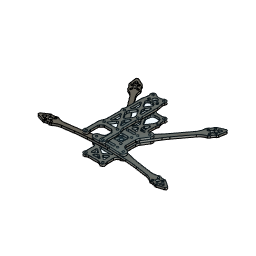
3inch Frame M3 v4 (Autodesk Fusion 360 design; units mm, degrees)
Autodesk Fusion 360 part; units mm, degrees
(part 1 of 3)
sketch "Skizze1" plane through (0, 0, 0) normal (0, 0, 1) x (1, 0, 0)
  line L0 (-8.4986, -15.4937) -> (8.4986, -15.4937)
  arc A0 (-5, -8.5) -> (-5, -11.5) centre (-5, -10) ccw
  line L1 (5.5, 1.5) -> (5.5, 8.5)
  arc A1 (-2.5, 11.5) -> (-5.5, 8.5) centre (-2.5, 8.5) ccw
  line L2 (9.0781, -17.3087) -> (1.159, -22.94)
  line L3 (-5, 18.5) -> (5, 18.5)
  arc A2 (5.5, 8.5) -> (2.5, 11.5) centre (2.5, 8.5) ccw
  line L4 (4.5469, -30.6788) -> (1.159, -28.2697)
  arc A3 (-16.0602, -5.4602) -> (-15.2136, -4.7566) centre (-25.2187, 6.4193) ccw
  line L5 (8.4205, -21.4575) -> (3.7344, -24.7899)
  line L6 (3.7344, -26.4198) -> (8.4205, -29.7522)
  circle A4 centre (12.5, -34.4937) radius 1
  arc A5 (-15.2136, -4.7566) -> (-13.8136, -1.2866) centre (-18.8136, -1.2866) ccw
  line L7 (5, 21.5) -> (-5, 21.5)
  arc A6 (1.159, -22.94) -> (-1.159, -22.94) centre (0, -21.3101) cw
  arc A7 (-9.6254, 27.8499) -> (-2.1571, 24.5) centre (-2.1571, 34.5) ccw
  line L8 (-5.5, 8.5) -> (-5.5, 1.5)
  circle A8 centre (-17.7913, 30.4065) radius 1
  arc A9 (11.2528, -36.6604) -> (8.7583, -35.9937) centre (8.7583, -40.9937) ccw
  line L9 (-5, -11.5) -> (5, -11.5)
  line L10 (-1.159, -28.2697) -> (-4.5469, -30.6788)
  arc A10 (2.5, -1.5) -> (5.5, 1.5) centre (2.5, 1.5) ccw
  line L11 (-1.159, -22.94) -> (-9.0781, -17.3087)
  arc A11 (1.159, -28.2697) -> (-1.159, -28.2697) centre (0, -29.8996) ccw
  arc A12 (-21.5229, 28.0783) -> (-14.5065, 33.3315) centre (-17.7913, 30.4065) cw
  arc A13 (-5.5, 1.5) -> (-2.5, -1.5) centre (-2.5, 1.5) ccw
  line L12 (-8.4205, -29.7522) -> (-3.7344, -26.4198)
  arc A14 (-10, -28.9372) -> (-8.4205, -29.7522) centre (-9, -28.9372) ccw
  line L13 (-15, -34.4937) -> (-15, -21.0235)
  line L14 (-13.8136, -1.2866) -> (-13.8136, 12.8582)
  arc A15 (5, -11.5) -> (5, -8.5) centre (5, -10) ccw
  line L15 (-14.5065, 33.3315) -> (-9.6254, 27.8499)
  line L16 (-2.5, -1.5) -> (2.5, -1.5)
  line L17 (5, -8.5) -> (-5, -8.5)
  arc A16 (3.9674, -32.4937) -> (4.5469, -30.6788) centre (3.9674, -31.4937) ccw
  line L18 (-3.9674, -32.4937) -> (3.9674, -32.4937)
  arc A17 (8.4986, -15.4937) -> (9.0781, -17.3087) centre (8.4986, -16.4937) cw
  line L19 (-3.7344, -24.7899) -> (-8.4205, -21.4575)
  arc A18 (-9.0781, -17.3087) -> (-8.4986, -15.4937) centre (-8.4986, -16.4937) cw
  line L20 (15, -21.0235) -> (15, -34.4937)
  arc A19 (19.9477, -16.0238) -> (15, -21.0235) centre (20, -21.0235) ccw
  arc A20 (8.4205, -29.7522) -> (10, -28.9372) centre (9, -28.9372) ccw
  line L21 (2.5, 11.5) -> (-2.5, 11.5)
  arc A21 (-4.5469, -30.6788) -> (-3.9674, -32.4937) centre (-3.9674, -31.4937) ccw
  arc A22 (15, -34.4937) -> (11.2528, -36.6604) centre (12.5, -34.4937) cw
  line L22 (13.8136, 12.8582) -> (13.8136, -1.2866)
  arc A23 (5, 18.5) -> (5, 21.5) centre (5, 20) ccw
  line L23 (-2.1571, 24.5) -> (2.1571, 24.5)
  circle A24 centre (-8, 13) radius 2
  arc A25 (15.3294, 18.1516) -> (13.8136, 12.8582) centre (23.8136, 12.8582) ccw
  circle A26 centre (-10, -10) radius 1
  arc A27 (10, -22.2725) -> (8.4205, -21.4575) centre (9, -22.2725) ccw
  circle A28 centre (19.8995, -11.4142) radius 1
  line L24 (8.7583, -35.9937) -> (-8.7583, -35.9937)
  line L25 (21.5229, 28.0783) -> (15.3294, 18.1516)
  arc A29 (-8.4205, -21.4575) -> (-10, -22.2725) centre (-9, -22.2725) ccw
  circle A30 centre (10, 20) radius 1
  arc A31 (-11.2528, -36.6604) -> (-15, -34.4937) centre (-12.5, -34.4937) cw
  arc A32 (-5, 21.5) -> (-5, 18.5) centre (-5, 20) ccw
  arc A33 (-3.7344, -26.4198) -> (-3.7344, -24.7899) centre (-4.3139, -25.6048) ccw
  arc A34 (-13.8136, 12.8582) -> (-15.3294, 18.1516) centre (-23.8136, 12.8582) ccw
  arc A35 (-17.6687, -6.1538) -> (-16.0602, -5.4602) centre (-18.8136, -1.2866) ccw
  line L26 (10, -28.9372) -> (10, -22.2725)
  arc A36 (20.9551, -6.9268) -> (19.9477, -16.0238) centre (19.8995, -11.4142) cw
  arc A37 (-8.7583, -35.9937) -> (-11.2528, -36.6604) centre (-8.7583, -40.9937) ccw
  circle A38 centre (8, 13) radius 2
  arc A39 (3.7344, -24.7899) -> (3.7344, -26.4198) centre (4.3139, -25.6048) ccw
  arc A40 (-15, -21.0235) -> (-19.9477, -16.0238) centre (-20, -21.0235) ccw
  arc A41 (-19.9477, -16.0238) -> (-20.9551, -6.9268) centre (-19.8995, -11.4142) cw
  arc A42 (15.2136, -4.7566) -> (16.0602, -5.4602) centre (25.2187, 6.4193) ccw
  circle A43 centre (10, -10) radius 1
  line L27 (9.6254, 27.8499) -> (14.5065, 33.3315)
  arc A44 (14.5065, 33.3315) -> (21.5229, 28.0783) centre (17.7913, 30.4065) cw
  line L28 (-15.3294, 18.1516) -> (-21.5229, 28.0783)
  circle A45 centre (-10, 20) radius 1
  circle A46 centre (8, -3) radius 2
  line L29 (17.6687, -6.1538) -> (20.9551, -6.9268)
  circle A47 centre (-19.8995, -11.4142) radius 1
  line L30 (-10, -22.2725) -> (-10, -28.9372)
  arc A48 (16.0602, -5.4602) -> (17.6687, -6.1538) centre (18.8136, -1.2866) ccw
  arc A49 (2.1571, 24.5) -> (9.6254, 27.8499) centre (2.1571, 34.5) ccw
  circle A50 centre (17.7913, 30.4065) radius 1
  circle A51 centre (-8, -3) radius 2
  arc A52 (13.8136, -1.2866) -> (15.2136, -4.7566) centre (18.8136, -1.2866) ccw
  circle A53 centre (-12.5, -34.4937) radius 1
  line L31 (-20.9551, -6.9268) -> (-17.6687, -6.1538)
extrude "Extrusion1" add sketch "Skizze1" along normal blind 3 makes body 1
sketch "Skizze2" plane through (0, 0, 0) normal (0, 0, 1) x (1, 0, 0)
  line L0 (50, -34.4937) -> (50, -19.2343)
  line L1 (25, -34.4937) -> (25, -14.0047)
  line L2 (28, 23.7417) -> (28, 48.0166)
  line L3 (28, 48.0166) -> (29.8264, 57.6051)
  arc A0 (30.5876, -17.771) -> (30, -19.187) centre (32, -19.187) ccw
  arc A1 (28, 16.2583) -> (27.3032, 18.6637) centre (23.5, 16.2583) ccw
  arc A2 (29.6382, 60.1802) -> (32.8799, 63.34) centre (32, 61) cw
  arc A3 (32.8799, 63.34) -> (33.9859, 62.9958) centre (36.3995, 72.7002) ccw
  arc A4 (46.584, -14.9827) -> (45.1731, -14.3952) centre (45.168, -16.3952) ccw
  arc A5 (34.8299, -14.3692) -> (33.4124, -14.9532) centre (34.8249, -16.3692) ccw
  line L4 (28, -3.4691) -> (28, 16.2583)
  arc A6 (37.582, 62.1014) -> (42.4175, 62.1034) centre (39.9957, 71.8057) ccw
  line L5 (42.4175, 62.1034) -> (46.0651, 63.0139)
  arc A7 (25, -14.0047) -> (26.5, -8.7369) centre (35, -14.0047) cw
  line L6 (45.1731, -14.3952) -> (34.8299, -14.3692)
  arc A8 (27.3032, 21.3363) -> (28, 23.7417) centre (23.5, 23.7417) ccw
  arc A9 (30, -34.4937) -> (25, -34.4937) centre (27.5, -34.4937) cw
  line L7 (33.9859, 62.9958) -> (37.582, 62.1014)
  arc A10 (27.3032, 18.6637) -> (27.3032, 21.3363) centre (29.4161, 20) cw
  line L8 (49.416, -17.8218) -> (46.584, -14.9827)
  arc A11 (52, -3.4691) -> (53.5, -8.7369) centre (62, -3.4691) ccw
  line L9 (37.0465, 33.3303) -> (37.0465, 35.9896)
  arc A12 (50, -19.2343) -> (49.416, -17.8218) centre (48, -19.2343) ccw
  line L10 (33.4124, -14.9532) -> (30.5876, -17.771)
  arc A13 (29.8264, 57.6051) -> (29.6382, 60.1802) centre (24.9147, 58.5407) ccw
  arc A14 (26.5, -8.7369) -> (28, -3.4691) centre (18, -3.4691) ccw
  line L11 (30, -19.187) -> (30, -34.4937)
  arc A15 (41.1255, 30.2175) -> (40.2838, 30.6775) centre (40.2838, 29.6775) ccw
  line L12 (34.1057, -9.3447) -> (45.9091, -9.3743)
  arc A16 (50.3618, 60.1802) -> (50.1736, 57.6051) centre (55.0853, 58.5407) ccw
  arc A17 (37.0465, 35.9896) -> (36.7299, 37.0695) centre (35.0465, 35.9896) ccw
  arc A18 (45.9091, -9.3743) -> (46.7436, -7.8196) centre (45.9116, -8.3743) ccw
  circle A19 centre (40, 56) radius 3.5
  arc A20 (33.3417, 42.3511) -> (31.5, 41.8112) centre (32.5, 41.8112) ccw
  arc A21 (36.3941, 50.4723) -> (38.2518, 50.7852) centre (37.6161, 48.889) cw
  arc A22 (52.6968, 18.6637) -> (52, 16.2583) centre (56.5, 16.2583) ccw
  line L13 (31.5, 38.4821) -> (31.6182, 27.626)
  arc A23 (38.2518, 50.7852) -> (41.7506, 50.7861) centre (40, 56) ccw
  arc A24 (45.3088, 49.1634) -> (45.7766, 46.5077) centre (44.0879, 47.5793) cw
  arc A25 (32.8235, 54.192) -> (34.7612, 54.3251) centre (33.8087, 54.0206) cw
  arc A26 (38.3359, 10.2003) -> (41.6641, 10.2003) centre (40, 11.3097) ccw
  arc A27 (39.8091, 38.6775) -> (38.9674, 39.1376) centre (39.8091, 39.6775) cw
  arc A28 (39.8347, 30.6775) -> (38.9903, 30.2133) centre (39.8347, 29.6775) ccw
  line L14 (45.7766, 46.5077) -> (41.1027, 39.1418)
  arc A29 (45.8881, 51.4617) -> (47.4838, 52.4251) centre (46.4986, 52.2538) ccw
  arc A30 (41.7506, 50.7861) -> (43.6082, 50.4741) centre (42.3872, 48.8901) cw
  circle A31 centre (50, -10) radius 1
  arc A32 (41.6641, -0.2003) -> (38.3359, -0.2003) centre (40, -1.3097) ccw
  arc A33 (33.2761, -7.79) -> (34.1057, -9.3447) centre (34.1082, -8.3447) ccw
  line L15 (46.168, 22.3571) -> (41.1255, 30.2175)
  arc A34 (46.0651, 63.0139) -> (47.1287, 63.3432) centre (43.6434, 72.7162) ccw
  arc A35 (36.7352, 32.2588) -> (37.0465, 33.3303) centre (35.0465, 33.3303) ccw
  line L16 (46.7436, -7.8196) -> (41.6641, -0.2003)
  line L17 (38.9903, 30.2133) -> (33.9075, 22.203)
  line L18 (34.7032, 49.1673) -> (36.3941, 50.4723)
  arc A36 (34.7612, 54.3251) -> (35.1808, 53.3495) centre (40, 56) ccw
  line L19 (52, 16.2583) -> (52, -3.4691)
  line L20 (38.3359, -0.2003) -> (33.2761, -7.79)
  arc A37 (33.9075, 22.203) -> (33.969, 16.7506) centre (38.1293, 19.5241) ccw
  line L21 (47.4838, 52.4251) -> (47.1765, 54.192)
  line L22 (52, 48.0166) -> (52, 23.7417)
  line L23 (33.969, 16.7506) -> (38.3359, 10.2003)
  line L24 (33.4625, 27.1011) -> (36.7352, 32.2588)
  line L25 (40.2838, 30.6775) -> (39.8347, 30.6775)
  arc A38 (35.1808, 53.3495) -> (34.9155, 52.076) centre (34.3046, 52.8676) cw
  line L26 (38.9674, 39.1376) -> (34.2418, 46.5041)
  line L27 (41.6641, 10.2003) -> (46.1198, 16.8839)
  line L28 (36.7299, 37.0695) -> (33.3417, 42.3511)
  arc A39 (34.2418, 46.5041) -> (34.7032, 49.1673) centre (35.9252, 47.584) cw
  arc A40 (47.1765, 54.192) -> (45.2388, 54.3251) centre (46.1913, 54.0206) ccw
  arc A41 (52, 23.7417) -> (52.6968, 21.3363) centre (56.5, 23.7417) ccw
  line L29 (55, -14.0047) -> (55, -34.4937)
  arc A42 (55, -34.4937) -> (50, -34.4937) centre (52.5, -34.4937) cw
  line L30 (43.6082, 50.4741) -> (45.3088, 49.1634)
  arc A43 (45.2388, 54.3251) -> (44.8209, 53.3526) centre (40, 56) cw
  arc A44 (53.5, -8.7369) -> (55, -14.0047) centre (45, -14.0047) cw
  arc A45 (52.6968, 21.3363) -> (52.6968, 18.6637) centre (50.5839, 20) cw
  line L31 (50.1736, 57.6051) -> (52, 48.0166)
  arc A46 (44.8209, 53.3526) -> (45.087, 52.0792) centre (45.6974, 52.8712) ccw
  line L32 (34.9155, 52.076) -> (34.1112, 51.4552)
  arc A47 (34.1112, 51.4552) -> (32.515, 52.4182) centre (33.5002, 52.2469) cw
  arc A48 (47.1287, 63.3432) -> (50.3618, 60.1802) centre (48, 61) cw
  line L33 (45.087, 52.0792) -> (45.8881, 51.4617)
  line L34 (32.515, 52.4182) -> (32.8235, 54.192)
  arc A49 (48.5, 11.7431) -> (46.6679, 12.2978) centre (47.5, 11.7431) ccw
  circle A50 centre (32, 61) radius 1
  arc A51 (31.5, -1.7431) -> (33.3321, -2.2978) centre (32.5, -1.7431) ccw
  line L35 (31.5, 11.7431) -> (31.5, -1.7431)
  arc A52 (46.6679, -2.2978) -> (48.5, -1.7431) centre (47.5, -1.7431) ccw
  line L36 (46.6556, 42.2937) -> (43.3578, 37.0963)
  arc A53 (43.3359, 7.2997) -> (43, 6.1903) centre (45, 6.1903) ccw
  line L37 (48.5, -1.7431) -> (48.5, 11.7431)
  arc A54 (43.3578, 37.0963) -> (43.0465, 36.0248) centre (45.0465, 36.0248) ccw
  arc A55 (46.1198, 16.8839) -> (46.168, 22.3571) centre (41.9595, 19.6574) ccw
  arc A56 (41.1027, 39.1418) -> (40.2583, 38.6775) centre (40.2583, 39.6775) cw
  line L38 (43.3359, 2.7003) -> (46.6679, -2.2978)
  line L39 (43, 6.1903) -> (43, 3.8097)
  arc A57 (31.6182, 27.626) -> (33.4625, 27.1011) centre (32.6182, 27.6369) ccw
  circle A58 centre (48, 61) radius 1
  circle A59 centre (30, 20) radius 1
  circle A60 centre (30, -10) radius 1
  line L40 (43.0465, 36.0248) -> (43.0465, 33.3654)
  circle A61 centre (50, 20) radius 1
  arc A62 (48.5, 41.7579) -> (46.6556, 42.2937) centre (47.5, 41.7579) ccw
  line L41 (36.6641, 7.2997) -> (33.3321, 12.2978)
  line L42 (31.5, 41.8112) -> (31.5, 38.4821)
  arc A63 (36.6641, 2.7003) -> (37, 3.8097) centre (35, 3.8097) ccw
  circle A64 centre (27.5, -34.4937) radius 1
  line L43 (43.3631, 32.2855) -> (46.6583, 27.1489)
  line L44 (37, 3.8097) -> (37, 6.1903)
  arc A65 (33.3321, 12.2978) -> (31.5, 11.7431) centre (32.5, 11.7431) ccw
  line L45 (46.6679, 12.2978) -> (43.3359, 7.2997)
  line L46 (33.3321, -2.2978) -> (36.6641, 2.7003)
  line L47 (48.5, 27.6888) -> (48.5, 41.7579)
  arc A66 (37, 6.1903) -> (36.6641, 7.2997) centre (35, 6.1903) ccw
  arc A67 (43.0465, 33.3654) -> (43.3631, 32.2855) centre (45.0465, 33.3654) ccw
  arc A68 (43, 3.8097) -> (43.3359, 2.7003) centre (45, 3.8097) ccw
  arc A69 (46.6583, 27.1489) -> (48.5, 27.6888) centre (47.5, 27.6888) ccw
  line L48 (40.2583, 38.6775) -> (39.8091, 38.6775)
  circle A70 centre (52.5, -34.4937) radius 1
extrude "Extrusion2" add sketch "Skizze2" along normal blind 3 separate body makes body 2
sketch "Skizze3" plane through (0, 0, 0) normal (0, 0, 1) x (1, 0, 0)
  line L0 (4.8, 8.9) -> (2.0164, 10.9877)
  arc A0 (-61.8005, -59.2444) -> (-59.2651, -61.785) centre (-59.9079, -59.8911) ccw
  line L1 (-51.05, -45.5) -> (-51.05, -44)
  arc A1 (-51.05, -44) -> (-48.95, -44) centre (-50, -44) cw
  line L2 (-48.95, -44) -> (-48.95, -45.5)
  line L3 (-14.4838, -19.2759) -> (-1.1141, -8.0998)
  arc A2 (-57.0625, -47.737) -> (-54.2422, -45.7569) centre (-61.3125, -38.6851) ccw
  arc A3 (1.8, 4.9) -> (4.2, 3.1) centre (3, 4) ccw
  arc A4 (-28.4671, -24.235) -> (-16.4086, -11.0537) centre (-169.857, 117.2178) ccw
  arc A5 (-57.0625, -47.737) -> (-58.3657, -49.1917) centre (-56, -50) ccw
  arc A6 (-36.0938, -40.3312) -> (-41.5498, -50.4967) centre (-21.9485, -54.4702) ccw
  arc A7 (-14.4838, -19.2759) -> (-21.0744, -25.3052) centre (49.652, -96.0001) ccw
  arc A8 (-42.9375, -52.263) -> (-45.7578, -54.2431) centre (-38.6875, -61.3149) ccw
  arc A9 (-45.7578, -54.2431) -> (-47.737, -57.0625) centre (-38.6851, -61.3125) ccw
  line L4 (9.6, 5.3) -> (7.2, 7.1)
  line L5 (-56, -48.95) -> (-54.5, -48.95)
  line L6 (-28.4671, -24.235) -> (-40.3312, -36.0938)
  arc A10 (-49.1964, -58.3673) -> (-47.737, -57.0625) centre (-50, -56) ccw
  line L7 (7.2, 7.1) -> (4.2, 3.1)
  line L8 (2.0164, 10.9877) -> (-16.4086, -11.0537)
  line L9 (-36.0938, -40.3312) -> (-21.0744, -25.3052)
  arc A11 (-50.4967, -41.5498) -> (-40.3312, -36.0938) centre (-54.4702, -21.9485) ccw
  arc A12 (-42.9375, -52.263) -> (-41.5498, -50.4967) centre (-44, -50) ccw
  line L10 (2.0588, -4.755) -> (9.6, 5.3)
  arc A13 (-58.0382, -56.6514) -> (-56.8125, -57.9074) centre (-57.0821, -56.9444) ccw
  line L11 (1.8, 4.9) -> (4.8, 8.9)
  arc A14 (-48.95, -45.5) -> (-51.05, -45.5) centre (-50, -45.5) cw
  line L12 (-56.995, -53.2471) -> (-58.0382, -56.6514)
  arc A15 (-45.5, -51.05) -> (-45.5, -48.95) centre (-45.5, -50) cw
  line L13 (-45.5, -48.95) -> (-44, -48.95)
  line L14 (-58.3657, -49.1917) -> (-61.8005, -59.2444)
  circle A16 centre (0, 0) radius 1
  line L15 (-54.5, -51.05) -> (-56, -51.05)
  line L16 (-56.8125, -57.9074) -> (-53.3687, -56.9432)
  line L17 (-51.05, -54.5) -> (-51.05, -56)
  arc A17 (-1.1141, -8.0998) -> (2.0588, -4.755) centre (-13.9412, 7.245) ccw
  circle A18 centre (-50, -50) radius 2.5
  arc A19 (-51.05, -56) -> (-48.95, -56) centre (-50, -56) ccw
  arc A20 (-53.3687, -56.9432) -> (-53.1185, -55.1259) centre (-53.6383, -55.9802) ccw
  arc A21 (-48.95, -54.5) -> (-51.05, -54.5) centre (-50, -54.5) ccw
  line L18 (-59.2651, -61.785) -> (-49.1964, -58.3673)
  circle A22 centre (-7.0711, -7.0711) radius 1
  arc A23 (-56, -48.95) -> (-56, -51.05) centre (-56, -50) ccw
  arc A24 (-54.2422, -45.7569) -> (-52.263, -42.9375) centre (-61.3149, -38.6875) ccw
  line L19 (-44, -51.05) -> (-45.5, -51.05)
  arc A25 (-55.1762, -53.0343) -> (-56.995, -53.2471) centre (-56.0389, -53.54) ccw
  arc A26 (-50.4967, -41.5498) -> (-52.263, -42.9375) centre (-50, -44) ccw
  arc A27 (-44, -48.95) -> (-44, -51.05) centre (-44, -50) cw
  arc A28 (-53.1185, -55.1259) -> (-55.1762, -53.0343) centre (-50, -50) cw
  line L20 (-48.95, -56) -> (-48.95, -54.5)
  arc A29 (-54.5, -51.05) -> (-54.5, -48.95) centre (-54.5, -50) ccw
extrude "Extrusion3" add sketch "Skizze3" along normal blind 3 separate body makes body 3
move_body "Verschieben1" bodies 3 to x (1, 0, 0) y (0, 1, 0) z (0, 0, 1) at (-35.6386, 44.251, 0)
copy_body "Körper kopieren/einfügen1" bodies 3 makes body 4
move_body "Verschieben2" bodies 4 to x (1, 0, 0) y (0, 1, 0) z (0, 0, 1) at (0.9596, -26.2227, 0)
sketch "Skizze4" plane through (0, 0, 0) normal (0, 0, 1) x (1, 0, 0)
  arc A0 (-51.8235, -55.2725) -> (-51.8231, -57.3725) centre (-51.8233, -56.3225) ccw
  arc A1 (2.8859, -4.961) -> (-1.6285, -6.6642) centre (2.1746, -9.9101) ccw
  line L0 (-57.3725, -60.8235) -> (-57.3722, -62.3235)
  line L1 (-63.0539, -64.2947) -> (-59.6319, -63.2926)
  line L2 (-60.8235, -55.2741) -> (-62.3235, -55.2744)
  line L3 (-4.761, -10.3344) -> (-1.6285, -6.6642)
  arc A2 (-62.3235, -55.2744) -> (-62.3231, -57.3744) centre (-62.3233, -56.3244) ccw
  arc A3 (-57.3722, -62.3235) -> (-55.2722, -62.3231) centre (-56.3222, -62.3233) ccw
  line L4 (-57.3744, -50.3235) -> (-57.3741, -51.8235)
  arc A4 (-57.3741, -51.8235) -> (-55.2741, -51.8231) centre (-56.3241, -51.8233) ccw
  arc A5 (-64.2946, -63.0539) -> (-63.0539, -64.2947) centre (-63.3349, -63.335) ccw
  line L5 (-62.3231, -57.3744) -> (-60.8231, -57.3741)
  arc A6 (-50.3231, -57.3722) -> (-50.3235, -55.2722) centre (-50.3233, -56.3222) ccw
  line L6 (-63.2923, -59.6322) -> (-64.2946, -63.0539)
  line L7 (-55.2722, -62.3231) -> (-55.2725, -60.8231)
  circle A7 centre (-9.1924, -9.1924) radius 1
  arc A8 (-60.8231, -57.3741) -> (-60.8235, -55.2741) centre (-60.8233, -56.3241) ccw
  arc A9 (-59.6319, -63.2926) -> (-59.4001, -61.4744) centre (-59.9129, -62.3329) ccw
  arc A10 (-55.2725, -60.8231) -> (-57.3725, -60.8235) centre (-56.3225, -60.8233) ccw
  line L8 (-55.2741, -51.8231) -> (-55.2744, -50.3231)
  circle A11 centre (0, 0) radius 1
  arc A12 (-10.5603, -16.0991) -> (-4.761, -10.3344) centre (-42.7923, 22.1252) ccw
  line L9 (2.8859, -4.961) -> (9.2582, -5.8767)
  line L10 (-51.8231, -57.3725) -> (-50.3231, -57.3722)
  circle A13 centre (-56.3233, -56.3233) radius 2.5
  line L11 (9.2582, -5.8767) -> (9.6849, -2.9072)
  line L12 (-50.3235, -55.2722) -> (-51.8235, -55.2725)
  arc A14 (-55.2744, -50.3231) -> (-57.3744, -50.3235) centre (-56.3244, -50.3233) ccw
  arc A15 (-0.252, 4.5824) -> (-4.7857, 2.8565) centre (-0.9633, -0.3667) ccw
  arc A16 (-59.4001, -61.4744) -> (-61.4741, -59.4005) centre (-56.3233, -56.3233) cw
  arc A17 (-41.7921, -46.0304) -> (-47.3656, -56.8241) centre (-27.6475, -60.17) ccw
  line L13 (9.6849, -2.9072) -> (4.7358, -2.196)
  line L14 (-65.668, -68.1443) -> (-55.49, -65.2056)
  arc A18 (-63.6367, -53.6272) -> (-65.2055, -55.492) centre (-62.3233, -56.3244) ccw
  arc A19 (-56.826, -47.3655) -> (-46.0299, -41.7916) centre (-60.1696, -27.647) ccw
  line L15 (10.1117, 0.0623) -> (10.5384, 3.0317)
  arc A20 (-55.49, -65.2056) -> (-53.6245, -63.6357) centre (-56.3222, -62.3233) ccw
  line L16 (-26.1459, -21.9145) -> (-46.0299, -41.7916)
  arc A21 (-61.4741, -59.4005) -> (-63.2923, -59.6322) centre (-62.3326, -59.9134) ccw
  arc A22 (-15.6554, -20.3955) -> (-21.9145, -26.1459) centre (48.8085, -96.8442) ccw
  arc A23 (-63.6367, -53.6272) -> (-59.0221, -49.011) centre (-68.0145, -44.6364) ccw
  line L17 (10.5384, 3.0317) -> (-0.252, 4.5824)
  line L18 (-4.7857, 2.8565) -> (-20.3955, -15.6554)
  arc A24 (-68.1443, -65.6679) -> (-65.668, -68.1443) centre (-66.2228, -66.2228) ccw
  line L19 (5.1625, 0.7735) -> (10.1117, 0.0623)
  line L20 (-15.6554, -20.3955) -> (-10.5603, -16.0991)
  arc A25 (-26.1459, -21.9145) -> (-20.3955, -15.6554) centre (-96.8442, 48.8085) ccw
  line L21 (-41.7921, -46.0304) -> (-21.9145, -26.1459)
  arc A26 (5.1625, 0.7735) -> (4.7358, -2.196) centre (4.9492, -0.7112) ccw
  arc A27 (-49.01, -59.0195) -> (-53.6245, -63.6357) centre (-44.6321, -68.0103) ccw
  line L22 (-65.2055, -55.492) -> (-68.1443, -65.6679)
  arc A28 (-56.826, -47.3655) -> (-59.0221, -49.011) centre (-56.3244, -50.3233) ccw
  arc A29 (-49.01, -59.0195) -> (-47.3656, -56.8241) centre (-50.3233, -56.3222) ccw
extrude "Extrusion4" add sketch "Skizze4" along normal blind 3 separate body makes body 5
move_body "Verschieben3" bodies 5 to x (1, 0, 0) y (0, 1, 0) z (0, 0, 1) at (-40.1263, -23.4528, 0)
copy_body "Körper kopieren/einfügen2" bodies 5 makes body 6
move_body "Verschieben4" bodies 6 to x (1, 0, 0) y (0, 1, 0) z (0, 0, 1) at (11.1608, -16.7575, 0)
sketch "Skizze5" plane through (0, 0, 0) normal (0, 0, 1) x (1, 0, 0)
  line L0 (-0.1909, 38.6775) -> (0.1909, 38.6775)
  arc A0 (5, 18.5) -> (5, 21.5) centre (5, 20) ccw
  arc A1 (14.5065, 33.3315) -> (21.5229, 28.0783) centre (17.7913, 30.4065) cw
  arc A2 (-5, 21.5) -> (-5, 18.5) centre (-5, 20) ccw
  arc A3 (-13.8136, 12.8582) -> (-15.3294, 18.1516) centre (-23.8136, 12.8582) ccw
  line L1 (-2.9535, 33.3303) -> (-2.9535, 35.9896)
  arc A4 (-14.1202, 32.8977) -> (-11.5, 33.8952) centre (-13, 33.8952) ccw
  arc A5 (-3.2648, 32.2588) -> (-2.9535, 33.3303) centre (-4.9535, 33.3303) ccw
  arc A6 (10.3618, 60.1802) -> (10.1736, 57.6051) centre (15.0853, 58.5407) ccw
  circle A7 centre (-10, 49.5) radius 1
  line L2 (-7.5, 30.5662) -> (-7.5, 29.0266)
  arc A8 (7.1025, 63.3333) -> (10.3618, 60.1802) centre (8, 61) cw
  line L3 (-5.3074, 63) -> (5.3074, 63)
  arc A9 (15.3294, 18.1516) -> (13.8136, 12.8582) centre (23.8136, 12.8582) ccw
  arc A10 (-11.5, 45.7583) -> (-12.1667, 48.2528) centre (-16.5, 45.7583) ccw
  arc A11 (5.3074, 63) -> (7.1025, 63.3333) centre (5.3074, 68) ccw
  line L4 (-20.9551, -6.9268) -> (-17.6687, -6.1538)
  arc A12 (11.9779, 51.0291) -> (12.1667, 48.2528) centre (10, 49.5) cw
  line L5 (19.6564, -16.0177) -> (2.637, -15.1188)
  arc A13 (-7.1025, 63.3333) -> (-5.3074, 63) centre (-5.3074, 68) ccw
  arc A14 (-12.1667, 48.2528) -> (-11.9779, 51.0291) centre (-10, 49.5) cw
  line L6 (-15.3294, 18.1516) -> (-21.5229, 28.0783)
  arc A15 (-19.6564, -16.0177) -> (-20.9551, -6.9268) centre (-19.8995, -11.4142) cw
  line L7 (-11.5, 33.8952) -> (-11.5, 45.7583)
  line L8 (3.6605, 26.0358) -> (1.0097, 30.2133)
  circle A16 centre (-8, 61) radius 1
  arc A17 (-3.5, 11.5) -> (-6.5, 8.5) centre (-3.5, 8.5) ccw
  arc A18 (13.8136, -1.2866) -> (17.6687, -6.1538) centre (18.8136, -1.2866) ccw
  line L9 (-5, 18.5) -> (5, 18.5)
  arc A19 (-17.6687, -6.1538) -> (-13.8136, -1.2866) centre (-18.8136, -1.2866) ccw
  arc A20 (-5, -8.5) -> (-5, -11.5) centre (-5, -10) ccw
  line L10 (0.1653, 30.6775) -> (-0.1653, 30.6775)
  arc A21 (-10.3618, 60.1802) -> (-7.1025, 63.3333) centre (-8, 61) cw
  arc A22 (-3.6605, 26.0358) -> (-2.8161, 24.5) centre (-2.8161, 25.5) ccw
  line L11 (-5.6556, 28.4909) -> (-3.2648, 32.2588)
  arc A23 (-2.9535, 35.9896) -> (-3.2701, 37.0695) centre (-4.9535, 35.9896) ccw
  line L12 (-13.8136, -1.2866) -> (-13.8136, 12.8582)
  line L13 (-2.637, -15.1188) -> (-19.6564, -16.0177)
  arc A24 (2.637, -15.1188) -> (-2.637, -15.1188) centre (0, -65.0492) ccw
  arc A25 (-11.9779, 51.0291) -> (-11.0219, 53.1517) centre (-15.9336, 54.0872) ccw
  line L14 (-14.5065, 33.3315) -> (-14.1202, 32.8977)
  arc A26 (-10.1736, 57.6051) -> (-10.3618, 60.1802) centre (-15.0853, 58.5407) ccw
  arc A27 (11.0219, 53.1517) -> (11.9779, 51.0291) centre (15.9336, 54.0872) ccw
  line L15 (10.1736, 57.6051) -> (11.0219, 53.1517)
  arc A28 (-21.5229, 28.0783) -> (-14.5065, 33.3315) centre (-17.7913, 30.4065) cw
  arc A29 (-6.1583, 41.5717) -> (-8, 41.0317) centre (-7, 41.0317) ccw
  line L16 (-11.0219, 53.1517) -> (-10.1736, 57.6051)
  line L17 (13.8136, 12.8582) -> (13.8136, -1.2866)
  arc A30 (20.9551, -6.9268) -> (19.6564, -16.0177) centre (19.8995, -11.4142) cw
  arc A31 (0.1909, 38.6775) -> (1.0326, 39.1376) centre (0.1909, 39.6775) ccw
  arc A32 (6.5, 8.5) -> (3.5, 11.5) centre (3.5, 8.5) ccw
  circle A33 centre (-8, -3) radius 1
  arc A34 (12.1667, 48.2528) -> (11.5, 45.7583) centre (16.5, 45.7583) ccw
  circle A35 centre (-10, 20) radius 1
  arc A36 (2.8161, 24.5) -> (3.6605, 26.0358) centre (2.8161, 25.5) ccw
  line L18 (-3.5, -1.5) -> (3.5, -1.5)
  line L19 (3.5, 11.5) -> (-3.5, 11.5)
  line L20 (17.6687, -6.1538) -> (20.9551, -6.9268)
  line L21 (-2.8161, 24.5) -> (2.8161, 24.5)
  line L22 (5, 21.5) -> (-5, 21.5)
  circle A37 centre (-17.7913, 30.4065) radius 1
  arc A38 (5, -11.5) -> (5, -8.5) centre (5, -10) ccw
  arc A39 (3.5, -1.5) -> (6.5, 1.5) centre (3.5, 1.5) ccw
  line L23 (2.9759, 59) -> (-2.9759, 59)
  circle A40 centre (-8, 13) radius 1
  arc A41 (11.5, 33.8952) -> (14.1202, 32.8977) centre (13, 33.8952) ccw
  line L24 (-5, -11.5) -> (5, -11.5)
  arc A42 (6.9168, 55.6854) -> (2.9759, 59) centre (2.9759, 55) ccw
  arc A43 (-2.9759, 59) -> (-6.9168, 55.6854) centre (-2.9759, 55) ccw
  arc A44 (-0.1653, 30.6775) -> (-1.0097, 30.2133) centre (-0.1653, 29.6775) ccw
  arc A45 (-7.7083, 31.5653) -> (-7.5, 30.5662) centre (-10, 30.5662) cw
  arc A46 (-7.5, 29.0266) -> (-5.6556, 28.4909) centre (-6.5, 29.0266) ccw
  line L25 (-6.9168, 55.6854) -> (-7.4589, 52.5682)
  line L26 (7.4589, 52.5682) -> (6.9168, 55.6854)
  circle A47 centre (-19.8995, -11.4142) radius 1
  line L27 (5, -8.5) -> (-5, -8.5)
  arc A48 (-6.5, 1.5) -> (-3.5, -1.5) centre (-3.5, 1.5) ccw
  line L28 (-6.5, 8.5) -> (-6.5, 1.5)
  line L29 (14.1202, 32.8977) -> (14.5065, 33.3315)
  line L30 (6.5, 1.5) -> (6.5, 8.5)
  line L31 (-1.0097, 30.2133) -> (-3.6605, 26.0358)
  circle A49 centre (-10, -10) radius 1
  line L32 (21.5229, 28.0783) -> (15.3294, 18.1516)
  line L33 (-8, 41.0317) -> (-8, 32.9641)
  circle A50 centre (-10, 29.5) radius 1
  arc A51 (1.0097, 30.2133) -> (0.1653, 30.6775) centre (0.1653, 29.6775) ccw
  line L34 (-3.2701, 37.0695) -> (-6.1583, 41.5717)
  arc A52 (-7.4589, 52.5682) -> (-6.4543, 47.5891) centre (-0.5624, 51.3688) ccw
  line L35 (-6.4543, 47.5891) -> (-1.0326, 39.1376)
  circle A53 centre (10, 29.5) radius 1
  line L36 (6.1583, 41.5717) -> (3.2701, 37.0695)
  circle A54 centre (8, 13) radius 1
  circle A55 centre (10, 20) radius 1
  line L37 (7.5, 29.0266) -> (7.5, 30.5662)
  arc A56 (3.2701, 37.0695) -> (2.9535, 35.9896) centre (4.9535, 35.9896) ccw
  circle A57 centre (8, 61) radius 1
  arc A58 (2.9535, 33.3303) -> (3.2648, 32.2588) centre (4.9535, 33.3303) ccw
  line L38 (3.2648, 32.2588) -> (5.6556, 28.4909)
  arc A59 (8, 41.0317) -> (6.1583, 41.5717) centre (7, 41.0317) ccw
  arc A60 (-1.0326, 39.1376) -> (-0.1909, 38.6775) centre (-0.1909, 39.6775) ccw
  circle A61 centre (10, 49.5) radius 1
  line L39 (11.5, 45.7583) -> (11.5, 33.8952)
  circle A62 centre (8, -3) radius 1
  arc A63 (7.5, 30.5662) -> (7.7083, 31.5653) centre (10, 30.5662) cw
  circle A64 centre (19.8995, -11.4142) radius 1
  arc A65 (7.7083, 31.5653) -> (8, 32.9641) centre (4.5, 32.9641) ccw
  circle A66 centre (10, -10) radius 1
  arc A67 (-8, 32.9641) -> (-7.7083, 31.5653) centre (-4.5, 32.9641) ccw
  line L40 (2.9535, 35.9896) -> (2.9535, 33.3303)
  line L41 (1.0326, 39.1376) -> (6.4543, 47.5891)
  arc A68 (6.4543, 47.5891) -> (7.4589, 52.5682) centre (0.5624, 51.3688) ccw
  line L42 (8, 32.9641) -> (8, 41.0317)
  arc A69 (5.6556, 28.4909) -> (7.5, 29.0266) centre (6.5, 29.0266) ccw
  circle A70 centre (17.7913, 30.4065) radius 1
extrude "Extrusion5" add sketch "Skizze5" along normal blind 3 separate body makes body 7
copy_body "Körper->Berechn1" bodies 1 removing the originals makes body 8 in component "Component"
copy_body "Körper->Berechn2" bodies 2 removing the originals makes body 9 in component "Component'"
copy_body "Körper->Berechn3" bodies 3 removing the originals makes body 10 in component "Component''"
copy_body "Körper->Berechn4" bodies 4 removing the originals makes body 11 in component "Component'''"
copy_body "Körper->Berechn5" bodies 5 removing the originals makes body 12 in component "Component''''"
copy_body "Körper->Berechn6" bodies 7 removing the originals makes body 13 in component "Component'''''"
copy_body "Körper->Berechn7" bodies 6 removing the originals makes body 14 in component "Component''''''"
sketch "Skizze14" plane through (0, 0, 6) normal (0, 0, -1) x (1, 0, 0)
  circle A0 centre (-22.8868, 11.6198) radius 1
  arc A1 (0.7471, 26.6254) -> (0.7471, 24.9955) centre (1.3266, 25.8105) ccw
  line L0 (0.7471, 26.6254) -> (5.4332, 29.9578)
  arc A2 (7.0127, 29.1428) -> (5.4332, 29.9578) centre (6.0127, 29.1428) ccw
  line L1 (7.0127, 29.1428) -> (7.0127, 22.4781)
  arc A3 (5.4332, 21.6632) -> (7.0127, 22.4781) centre (6.0127, 22.4781) ccw
  line L2 (5.4332, 21.6632) -> (0.7471, 24.9955)
  circle A4 centre (-10.9873, -12.7944) radius 2
  circle A5 centre (-10.9873, 3.2056) radius 2
  line L3 (2.0127, 8.7056) -> (-7.9873, 8.7056)
  arc A6 (-7.9873, 11.7056) -> (-7.9873, 8.7056) centre (-7.9873, 10.2056) ccw
  line L4 (-7.9873, 11.7056) -> (2.0127, 11.7056)
  arc A7 (2.0127, 8.7056) -> (2.0127, 11.7056) centre (2.0127, 10.2056) ccw
  arc A8 (-6.9546, 32.6994) -> (-7.5342, 30.8844) centre (-6.9546, 31.6994) ccw
  line L5 (-6.9546, 32.6994) -> (0.9801, 32.6994)
  arc A9 (1.5596, 30.8844) -> (0.9801, 32.6994) centre (0.9801, 31.6994) ccw
  line L6 (1.5596, 30.8844) -> (-1.8282, 28.4753)
  arc A10 (-4.1463, 28.4753) -> (-1.8282, 28.4753) centre (-2.9873, 30.1052) ccw
  line L7 (-4.1463, 28.4753) -> (-7.5342, 30.8844)
  circle A11 centre (7.0127, -19.7944) radius 1
  circle A12 centre (9.5127, 34.6994) radius 1
  circle A13 centre (-12.9873, -19.7944) radius 1
  circle A14 centre (5.0127, -12.7944) radius 2
  line L8 (-12.9873, 22.4781) -> (-12.9873, 29.1428)
  arc A15 (-11.4077, 29.9578) -> (-12.9873, 29.1428) centre (-11.9873, 29.1428) ccw
  line L9 (-11.4077, 29.9578) -> (-6.7216, 26.6254)
  arc A16 (-6.7216, 24.9955) -> (-6.7216, 26.6254) centre (-7.3012, 25.8105) ccw
  line L10 (-6.7216, 24.9955) -> (-11.4077, 21.6632)
  arc A17 (-12.9873, 22.4781) -> (-11.4077, 21.6632) centre (-11.9873, 22.4781) ccw
  arc A18 (-7.9873, -18.2944) -> (-7.9873, -21.2944) centre (-7.9873, -19.7944) ccw
  line L11 (-7.9873, -18.2944) -> (2.0127, -18.2944)
  arc A19 (2.0127, -21.2944) -> (2.0127, -18.2944) centre (2.0127, -19.7944) ccw
  line L12 (2.0127, -21.2944) -> (-7.9873, -21.2944)
  circle A20 centre (7.0127, 10.2056) radius 1
  circle A21 centre (14.804, -30.2009) radius 1
  circle A22 centre (-15.4873, 34.6994) radius 1
  circle A23 centre (5.0127, 3.2056) radius 2
  line L13 (-12.0654, 17.5143) -> (-4.1463, 23.1457)
  arc A24 (-1.8282, 23.1457) -> (-4.1463, 23.1457) centre (-2.9873, 21.5158) ccw
  line L14 (-1.8282, 23.1457) -> (6.0909, 17.5143)
  arc A25 (5.5113, 15.6994) -> (6.0909, 17.5143) centre (5.5113, 16.6994) ccw
  line L15 (5.5113, 15.6994) -> (-11.4859, 15.6994)
  arc A26 (-12.0654, 17.5143) -> (-11.4859, 15.6994) centre (-11.4859, 16.6994) ccw
  circle A27 centre (16.9122, 11.6198) radius 1
  circle A28 centre (-12.9873, 10.2056) radius 1
  line L16 (-0.4873, -11.2944) -> (-5.4873, -11.2944)
  arc A29 (-8.4873, -8.2944) -> (-5.4873, -11.2944) centre (-5.4873, -8.2944) ccw
  line L17 (-8.4873, -8.2944) -> (-8.4873, -1.2944)
  arc A30 (-5.4873, 1.7056) -> (-8.4873, -1.2944) centre (-5.4873, -1.2944) ccw
  line L18 (-5.4873, 1.7056) -> (-0.4873, 1.7056)
  arc A31 (2.5127, -1.2944) -> (-0.4873, 1.7056) centre (-0.4873, -1.2944) ccw
  line L19 (2.5127, -1.2944) -> (2.5127, -8.2944)
  arc A32 (-0.4873, -11.2944) -> (2.5127, -8.2944) centre (-0.4873, -8.2944) ccw
  circle A33 centre (-20.7786, -30.2009) radius 1
  arc A34 (-22.935, 16.2294) -> (-23.9423, 7.1324) centre (-22.8868, 11.6198) ccw
  line L20 (-23.9423, 7.1324) -> (-20.6559, 6.3594)
  arc A35 (-19.0475, 5.6658) -> (-20.6559, 6.3594) centre (-21.8008, 1.4922) ccw
  arc A36 (-18.2009, 4.9622) -> (-19.0475, 5.6658) centre (-28.2059, -6.2137) ccw
  arc A37 (-16.8008, 1.4922) -> (-18.2009, 4.9622) centre (-21.8008, 1.4922) ccw
  line L21 (-16.8008, 1.4922) -> (-16.8008, -12.6526)
  arc A38 (-18.3167, -17.946) -> (-16.8008, -12.6526) centre (-26.8008, -12.6526) ccw
  line L22 (-18.3167, -17.946) -> (-24.5102, -27.8727)
  arc A39 (-24.5102, -27.8727) -> (-17.4938, -33.1258) centre (-20.7786, -30.2009) ccw
  line L23 (-17.4938, -33.1258) -> (-12.6127, -27.6442)
  arc A40 (-5.1444, -24.2944) -> (-12.6127, -27.6442) centre (-5.1444, -34.2944) ccw
  line L24 (-5.1444, -24.2944) -> (-0.8301, -24.2944)
  arc A41 (6.6382, -27.6442) -> (-0.8301, -24.2944) centre (-0.8301, -34.2944) ccw
  line L25 (6.6382, -27.6442) -> (11.5192, -33.1258)
  arc A42 (11.5192, -33.1258) -> (18.5356, -27.8727) centre (14.804, -30.2009) ccw
  line L26 (18.5356, -27.8727) -> (12.3422, -17.946)
  arc A43 (10.8263, -12.6526) -> (12.3422, -17.946) centre (20.8263, -12.6526) ccw
  line L27 (10.8263, -12.6526) -> (10.8263, 1.4922)
  arc A44 (12.2264, 4.9622) -> (10.8263, 1.4922) centre (15.8263, 1.4922) ccw
  arc A45 (13.0729, 5.6658) -> (12.2264, 4.9622) centre (22.2314, -6.2137) ccw
  arc A46 (14.6814, 6.3594) -> (13.0729, 5.6658) centre (15.8263, 1.4922) ccw
  line L28 (14.6814, 6.3594) -> (17.9678, 7.1324)
  arc A47 (17.9678, 7.1324) -> (16.9604, 16.2294) centre (16.9122, 11.6198) ccw
  arc A48 (12.0127, 21.2292) -> (16.9604, 16.2294) centre (17.0127, 21.2292) ccw
  line L29 (12.0127, 21.2292) -> (12.0127, 34.6994)
  arc A49 (12.0127, 34.6994) -> (8.2655, 36.866) centre (9.5127, 34.6994) ccw
  arc A50 (5.7711, 36.1994) -> (8.2655, 36.866) centre (5.7711, 41.1994) ccw
  line L30 (5.7711, 36.1994) -> (-11.7456, 36.1994)
  arc A51 (-14.2401, 36.866) -> (-11.7456, 36.1994) centre (-11.7456, 41.1994) ccw
  arc A52 (-14.2401, 36.866) -> (-17.9873, 34.6994) centre (-15.4873, 34.6994) ccw
  line L31 (-17.9873, 34.6994) -> (-17.9873, 21.2292)
  arc A53 (-22.935, 16.2294) -> (-17.9873, 21.2292) centre (-22.9873, 21.2292) ccw
  circle A54 centre (-20.7786, -30.2009) radius 1.5
  circle A55 centre (14.804, -30.2009) radius 1.5
  circle A56 centre (-12.9873, -19.7944) radius 1.5
  circle A57 centre (7.0127, -19.7944) radius 1.5
  circle A58 centre (-22.8868, 11.6198) radius 1.5
  circle A59 centre (-12.9873, 10.2056) radius 1.5
  circle A60 centre (7.0127, 10.2056) radius 1.5
  circle A61 centre (16.9122, 11.6198) radius 1.5
  circle A62 centre (9.5127, 34.6994) radius 1.5
  circle A63 centre (-15.4873, 34.6994) radius 1.5
  circle A64 centre (-15.4873, 34.6994) radius 3.5
  circle A65 centre (9.5127, 34.6994) radius 3.5
  circle A66 centre (-10.9873, -12.7944) radius 3
  circle A67 centre (-10.9873, 3.2056) radius 3
  circle A68 centre (5.0127, 3.2056) radius 3
  circle A69 centre (5.0127, -12.7944) radius 3
  dimension "d139" = 3
  dimension "d140" = 3
  dimension "d141" = 3
  dimension "d142" = 3
  dimension "d143" = 3
  dimension "d144" = 3
  dimension "d145" = 3
  dimension "d146" = 3
  dimension "d147" = 3
  dimension "d148" = 3
  dimension "d149" = 7
  dimension "d150" = 7
  dimension "d239" = 6
  dimension "d240" = 6
  dimension "d241" = 6
  dimension "d242" = 6
  constraint concentric A33 A54
  constraint concentric A21 A55
  constraint concentric A13 A56
  constraint concentric A11 A57
  constraint concentric A0 A58
  constraint concentric A28 A59
  constraint concentric A20 A60
  constraint concentric A27 A61
  constraint concentric A12 A62
  constraint concentric A22 A63
  constraint concentric A63 A64
  constraint concentric A62 A65
  constraint concentric A4 A66
  constraint concentric A5 A67
  constraint concentric A23 A68
  constraint concentric A14 A69
  measures "d139" diameter of A54
  measures "d140" diameter of A55
  measures "d141" diameter of A56
  measures "d142" diameter of A57
  measures "d143" diameter of A58
  measures "d144" diameter of A59
  measures "d145" diameter of A60
  measures "d146" diameter of A61
  measures "d147" diameter of A62
  measures "d148" diameter of A63
  measures "d149" diameter of A64
  measures "d150" diameter of A65
  measures "d239" diameter of A66
  measures "d240" diameter of A67
  measures "d241" diameter of A68
  measures "d242" diameter of A69
extrude "Extrusion1'" cut sketch "Skizze14" against normal blind 3 contours A54 | A55 | A56 | A57 | A58 | A59 | A60 | A61 | A62 | A63 | A66 | A67 | A68 | A69 sketch seen with x (1, 0, 0) y (0, 1, 0) z (0, 0, 1) at (2.9873, 0.2056, -6) bodies 8 in component "Component"
extrude "Extrusion2'" add sketch "Skizze14" against normal blind 3 contours A51 A52 L31 A64 | L29 A49 A50 A65 picked at (-13.718, 36.9499) picked at (7.7572, 36.9609) sketch seen with x (1, 0, 0) y (0, 1, 0) z (0, 0, 1) at (2.9873, 0.2056, -6) bodies 8 in component "Component"
fillet "Abrundung1" radius 5 4 edges at (15, -32.0442, 1.5) (9.3549, -36.0295, 1.5) (-9.3549, -36.0295, 1.5) (-15, -32.0442, 1.5) on bodies 8 in component "Component"
sketch "Skizze15" plane through (0, 0, -23) normal (0, 0, -1) x (1, 0, 0)
  arc A0 (0.3486, -2.4947) -> (0.0127, -3.6041) centre (2.0127, -3.6041) ccw
  line L0 (0.3486, -2.4947) -> (3.6807, 2.5034)
  arc A1 (5.5127, 1.9487) -> (3.6807, 2.5034) centre (4.5127, 1.9487) ccw
  line L1 (5.5127, 1.9487) -> (5.5127, -11.5374)
  arc A2 (3.6807, -12.0921) -> (5.5127, -11.5374) centre (4.5127, -11.5374) ccw
  line L2 (3.6807, -12.0921) -> (0.3486, -7.0941)
  arc A3 (0.0127, -5.9847) -> (0.3486, -7.0941) centre (2.0127, -5.9847) ccw
  line L3 (0.0127, -5.9847) -> (0.0127, -3.6041)
  arc A4 (5.5127, -27.4832) -> (3.671, -26.9433) centre (4.5127, -27.4832) ccw
  line L4 (5.5127, -27.4832) -> (5.5127, -41.5523)
  arc A5 (3.6684, -42.088) -> (5.5127, -41.5523) centre (4.5127, -41.5523) ccw
  line L5 (3.6684, -42.088) -> (0.3705, -36.8907)
  arc A6 (0.0592, -35.8191) -> (0.3705, -36.8907) centre (2.0592, -35.8191) ccw
  line L6 (0.0592, -35.8191) -> (0.0592, -33.1598)
  arc A7 (0.3758, -32.0799) -> (0.0592, -33.1598) centre (2.0592, -33.1598) ccw
  line L7 (0.3758, -32.0799) -> (3.671, -26.9433)
  arc A8 (-1.8846, -38.9361) -> (-2.7289, -38.4719) centre (-2.7289, -39.4719) ccw
  line L8 (-1.8846, -38.9361) -> (2.7893, -46.3021)
  arc A9 (2.3216, -48.9577) -> (2.7893, -46.3021) centre (1.1006, -47.3737) ccw
  line L9 (2.3216, -48.9577) -> (0.6209, -50.2685)
  arc A10 (-1.2366, -50.5804) -> (0.6209, -50.2685) centre (-0.6, -48.6845) ccw
  arc A11 (-1.2366, -50.5804) -> (-4.7355, -50.5796) centre (-2.9873, -55.7944) ccw
  arc A12 (-6.5931, -50.2666) -> (-4.7355, -50.5796) centre (-5.3712, -48.6833) ccw
  line L10 (-6.5931, -50.2666) -> (-8.284, -48.9617)
  arc A13 (-8.7455, -46.2984) -> (-8.284, -48.9617) centre (-7.0621, -47.3784) ccw
  line L11 (-8.7455, -46.2984) -> (-4.0198, -38.932)
  arc A14 (-3.1781, -38.4719) -> (-4.0198, -38.932) centre (-3.1781, -39.4719) ccw
  line L12 (-3.1781, -38.4719) -> (-2.7289, -38.4719)
  circle A15 centre (-12.9873, 10.2056) radius 1
  arc A16 (-6.3232, -7.0941) -> (-5.9873, -5.9847) centre (-7.9873, -5.9847) ccw
  line L13 (-6.3232, -7.0941) -> (-9.6552, -12.0921)
  arc A17 (-11.4873, -11.5374) -> (-9.6552, -12.0921) centre (-10.4873, -11.5374) ccw
  line L14 (-11.4873, -11.5374) -> (-11.4873, 1.9487)
  arc A18 (-9.6552, 2.5034) -> (-11.4873, 1.9487) centre (-10.4873, 1.9487) ccw
  line L15 (-9.6552, 2.5034) -> (-6.3232, -2.4947)
  arc A19 (-5.9873, -3.6041) -> (-6.3232, -2.4947) centre (-7.9873, -3.6041) ccw
  line L16 (-5.9873, -3.6041) -> (-5.9873, -5.9847)
  circle A20 centre (9.5127, 34.6994) radius 1
  line L17 (-11.4873, -41.6055) -> (-11.4873, -38.2764)
  line L18 (-11.4873, -38.2764) -> (-11.369, -27.4204)
  arc A21 (-9.5247, -26.8955) -> (-11.369, -27.4204) centre (-10.3691, -27.4313) ccw
  line L19 (-9.5247, -26.8955) -> (-6.2521, -32.0531)
  arc A22 (-5.9408, -33.1247) -> (-6.2521, -32.0531) centre (-7.9408, -33.1247) ccw
  line L20 (-5.9408, -33.1247) -> (-5.9408, -35.784)
  arc A23 (-6.2574, -36.8639) -> (-5.9408, -35.784) centre (-7.9408, -35.784) ccw
  line L21 (-6.2574, -36.8639) -> (-9.6456, -42.1455)
  arc A24 (-11.4873, -41.6055) -> (-9.6456, -42.1455) centre (-10.4873, -41.6055) ccw
  circle A25 centre (-15.4873, 34.6994) radius 1
  circle A26 centre (7.0127, -19.7944) radius 1
  circle A27 centre (-12.9873, -19.7944) radius 1
  circle A28 centre (5.0127, -60.7944) radius 1
  circle A29 centre (-2.9873, -55.7944) radius 3.5
  circle A30 centre (7.0127, 10.2056) radius 1
  arc A31 (-8.8761, -51.2496) -> (-10.4723, -52.2126) centre (-9.487, -52.0412) ccw
  line L22 (-8.8761, -51.2496) -> (-8.0717, -51.8703)
  arc A32 (-7.8065, -53.1439) -> (-8.0717, -51.8703) centre (-8.6827, -52.662) ccw
  arc A33 (-7.8065, -53.1439) -> (-8.2261, -54.1195) centre (-2.9873, -55.7944) ccw
  arc A34 (-10.1638, -53.9863) -> (-8.2261, -54.1195) centre (-9.1786, -53.815) ccw
  line L23 (-10.1638, -53.9863) -> (-10.4723, -52.2126)
  line L24 (-4.6514, 0.4059) -> (-9.7111, 7.9956)
  arc A35 (-8.8816, 9.5503) -> (-9.7111, 7.9956) centre (-8.8791, 8.5503) ccw
  line L25 (-8.8816, 9.5503) -> (2.9218, 9.5799)
  arc A36 (3.7564, 8.0252) -> (2.9218, 9.5799) centre (2.9243, 8.5799) ccw
  line L26 (3.7564, 8.0252) -> (-1.3232, 0.4059)
  arc A37 (-4.6514, 0.4059) -> (-1.3232, 0.4059) centre (-2.9873, 1.5153) ccw
  line L27 (2.0997, -51.8736) -> (2.9008, -51.2561)
  arc A38 (4.4965, -52.2195) -> (2.9008, -51.2561) centre (3.5113, -52.0481) ccw
  line L28 (4.4965, -52.2195) -> (4.1892, -53.9863)
  arc A39 (2.2515, -54.1195) -> (4.1892, -53.9863) centre (3.204, -53.815) ccw
  arc A40 (2.2515, -54.1195) -> (1.8336, -53.147) centre (-2.9873, -55.7944) ccw
  arc A41 (2.0997, -51.8736) -> (1.8336, -53.147) centre (2.7102, -52.6656) ccw
  circle A42 centre (-10.9873, -60.7944) radius 1
  arc A43 (3.1807, -22.1515) -> (3.1325, -16.6782) centre (-1.0277, -19.4517) ccw
  line L29 (3.1807, -22.1515) -> (-1.8617, -30.0119)
  arc A44 (-2.7034, -30.4719) -> (-1.8617, -30.0119) centre (-2.7034, -29.4719) ccw
  line L30 (-2.7034, -30.4719) -> (-3.1526, -30.4719)
  arc A45 (-3.997, -30.0077) -> (-3.1526, -30.4719) centre (-3.1526, -29.4719) ccw
  line L31 (-3.997, -30.0077) -> (-9.0798, -21.9974)
  arc A46 (-9.0182, -16.545) -> (-9.0798, -21.9974) centre (-4.858, -19.3185) ccw
  line L32 (-9.0182, -16.545) -> (-4.6514, -9.9947)
  arc A47 (-1.3232, -9.9947) -> (-4.6514, -9.9947) centre (-2.9873, -11.1041) ccw
  line L33 (-1.3232, -9.9947) -> (3.1325, -16.6782)
  arc A48 (4.1414, -63.1376) -> (3.0779, -62.8083) centre (0.6561, -72.5106) ccw
  arc A49 (4.1414, -63.1376) -> (7.3745, -59.9746) centre (5.0127, -60.7944) ccw
  arc A50 (7.1863, -57.3995) -> (7.3745, -59.9746) centre (12.098, -58.335) ccw
  line L34 (7.1863, -57.3995) -> (9.0127, -47.811)
  line L35 (9.0127, -47.811) -> (9.0127, -23.536)
  arc A51 (9.7095, -21.1307) -> (9.0127, -23.536) centre (13.5127, -23.536) ccw
  arc A52 (9.7095, -21.1307) -> (9.7095, -18.4581) centre (7.5967, -19.7944) ccw
  arc A53 (9.0127, -16.0527) -> (9.7095, -18.4581) centre (13.5127, -16.0527) ccw
  line L36 (9.0127, -16.0527) -> (9.0127, 3.6747)
  arc A54 (10.5127, 8.9425) -> (9.0127, 3.6747) centre (19.0127, 3.6747) ccw
  arc A55 (10.5127, 8.9425) -> (12.0127, 14.2103) centre (2.0127, 14.2103) ccw
  line L37 (12.0127, 14.2103) -> (12.0127, 34.6994)
  arc A56 (12.0127, 34.6994) -> (7.0127, 34.6994) centre (9.5127, 34.6994) ccw
  line L38 (7.0127, 34.6994) -> (7.0127, 19.4399)
  arc A57 (6.4287, 18.0275) -> (7.0127, 19.4399) centre (5.0127, 19.4399) ccw
  line L39 (6.4287, 18.0275) -> (3.5968, 15.1884)
  arc A58 (2.1858, 14.6008) -> (3.5968, 15.1884) centre (2.1808, 16.6008) ccw
  line L40 (2.1858, 14.6008) -> (-8.1574, 14.5748)
  arc A59 (-9.5748, 15.1588) -> (-8.1574, 14.5748) centre (-8.1624, 16.5748) ccw
  line L41 (-9.5748, 15.1588) -> (-12.3997, 17.9766)
  arc A60 (-12.9873, 19.3926) -> (-12.3997, 17.9766) centre (-10.9873, 19.3926) ccw
  line L42 (-12.9873, 19.3926) -> (-12.9873, 34.6994)
  arc A61 (-12.9873, 34.6994) -> (-17.9873, 34.6994) centre (-15.4873, 34.6994) ccw
  line L43 (-17.9873, 34.6994) -> (-17.9873, 14.2103)
  arc A62 (-17.9873, 14.2103) -> (-16.4873, 8.9425) centre (-7.9873, 14.2103) ccw
  arc A63 (-14.9873, 3.6747) -> (-16.4873, 8.9425) centre (-24.9873, 3.6747) ccw
  line L44 (-14.9873, 3.6747) -> (-14.9873, -16.0527)
  arc A64 (-15.6841, -18.4581) -> (-14.9873, -16.0527) centre (-19.4873, -16.0527) ccw
  arc A65 (-15.6841, -18.4581) -> (-15.6841, -21.1307) centre (-13.5712, -19.7944) ccw
  arc A66 (-14.9873, -23.536) -> (-15.6841, -21.1307) centre (-19.4873, -23.536) ccw
  line L45 (-14.9873, -23.536) -> (-14.9873, -47.811)
  line L46 (-14.9873, -47.811) -> (-13.1609, -57.3995)
  arc A67 (-13.349, -59.9746) -> (-13.1609, -57.3995) centre (-18.0726, -58.335) ccw
  arc A68 (-13.349, -59.9746) -> (-10.1074, -63.1344) centre (-10.9873, -60.7944) ccw
  arc A69 (-9.0014, -62.7902) -> (-10.1074, -63.1344) centre (-6.5877, -72.4946) ccw
  line L47 (-9.0014, -62.7902) -> (-5.4052, -61.8958)
  arc A70 (-0.5698, -61.8978) -> (-5.4052, -61.8958) centre (-2.9916, -71.6001) ccw
  line L48 (-0.5698, -61.8978) -> (3.0779, -62.8083)
  circle A71 centre (-15.4873, 34.6994) radius 1.5
  circle A72 centre (9.5127, 34.6994) radius 1.5
  circle A73 centre (-12.9873, 10.2056) radius 1.5
  circle A74 centre (7.0127, 10.2056) radius 1.5
  circle A75 centre (-12.9873, -19.7944) radius 1.5
  circle A76 centre (7.0127, -19.7944) radius 1.5
  circle A77 centre (-10.9873, -60.7944) radius 1.5
  circle A78 centre (5.0127, -60.7944) radius 1.5
  circle A79 centre (-10.9873, -60.7944) radius 3.5
  circle A80 centre (5.0127, -60.7944) radius 3.5
  circle A81 centre (-12.9873, -19.7944) radius 3.5
  circle A82 centre (7.0127, -19.7944) radius 3.5
  circle A83 centre (9.5127, 34.6994) radius 3.5
  circle A84 centre (-15.4873, 34.6994) radius 3.5
  dimension "d157" = 3
  dimension "d158" = 3
  dimension "d159" = 3
  dimension "d160" = 3
  dimension "d161" = 3
  dimension "d162" = 3
  dimension "d163" = 3
  dimension "d164" = 3
  dimension "d165" = 7
  dimension "d166" = 7
  dimension "d167" = 7
  dimension "d168" = 7
  dimension "d169" = 7
  dimension "d170" = 7
  constraint concentric A25 A71
  constraint concentric A20 A72
  constraint concentric A15 A73
  constraint concentric A30 A74
  constraint concentric A27 A75
  constraint concentric A26 A76
  constraint concentric A42 A77
  constraint concentric A28 A78
  constraint concentric A77 A79
  constraint concentric A28 A80
  constraint concentric A75 A81
  constraint concentric A76 A82
  constraint concentric A72 A83
  constraint concentric A71 A84
  measures "d157" diameter of A71
  measures "d158" diameter of A72
  measures "d159" diameter of A73
  measures "d160" diameter of A74
  measures "d161" diameter of A75
  measures "d162" diameter of A76
  measures "d163" diameter of A77
  measures "d164" diameter of A78
  measures "d165" diameter of A79
  measures "d166" diameter of A80
  measures "d167" diameter of A81
  measures "d168" diameter of A82
  measures "d169" diameter of A83
  measures "d170" diameter of A84
extrude "Extrusion1''" cut sketch "Skizze15" against normal blind 3 contours A71 | A72 | A73 | A74 | A75 | A76 | A77 | A78 sketch seen with x (1, 0, 0) y (0, 1, 0) z (0, 0, 1) at (42.9873, 0.2056, 23) bodies 9 in component "Component'"
extrude "Extrusion2''" add sketch "Skizze15" against normal blind 3 contours A43 A82 | A51 A52 A53 A82 | A48 A49 A50 L48 A80 | A46 A81 | A64 A65 A66 A81 | L37 A56 L38 A83 | A67 A68 A69 L47 A79 | L42 A61 L43 A84 picked at (7.6038, -59.5802) picked at (7.1959, 36.8491) picked at (-13.5353, -59.489) picked at (-17.8041, 36.8491) sketch seen with x (1, 0, 0) y (0, 1, 0) z (0, 0, 1) at (42.9873, 0.2056, 23) bodies 9 in component "Component'"
fillet "Abrundung1'" radius 5 16 edges at (29.9029, 58.1978, 1.5) (35.0405, 62.7335, 1.5) (44.9624, 62.7386, 1.5) (50.0971, 58.1978, 1.5) (52.0996, 22.8003, 1.5) (52.0996, 17.1997, 1.5) (33.3531, 21.0033, 1.5) (33.2131, 18.6123, 1.5) (55, -32.0442, 1.5) (30, -32.0442, 1.5) (50, -32.0442, 1.5) (25, -32.0442, 1.5) (27.9004, 17.1997, 1.5) (46.8284, 18.5198, 1.5) (46.714, 21.205, 1.5) (27.9004, 22.8003, 1.5) on bodies 9 in component "Component'"